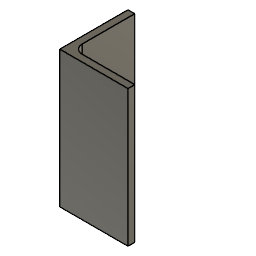
L-50×50×5 (Autodesk Fusion 360 design; units mm, degrees)
Autodesk Fusion 360 part; units mm, degrees
note: some values were not read from the file. Set by a fixed rule: which sketch regions a step uses.
sketch "スケッチ1" plane through (0, 0, 0) normal (0, 0, 1) x (1, 0, 0)
  line L0 (50, 5) -> (11.5, 5)
  line L1 (0, 0) -> (50, 0)
  line L2 (0, 50) -> (0, 0)
  line L3 (5, 11.5) -> (5, 50)
  arc A0 (5, 11.5) -> (11.5, 5) centre (11.5, 11.5) ccw
  line L4 (5, 50) -> (0, 50)
  line L5 (50, 0) -> (50, 5)
extrude "押し出し1" add sketch "スケッチ1" along normal blind 100
